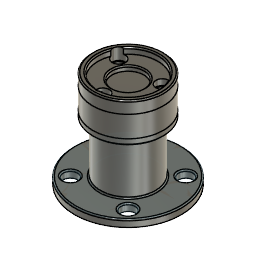
RV1-WHL-001_Wheel_Hub_Adapter (Autodesk Fusion 360 design; units mm, degrees)
part number: 2026-03-30-19-50-54-064
Autodesk Fusion 360 part; units mm, degrees
note: some values were not read from the file. Set by a fixed rule: which sketch regions a step uses.
sketch "Sketch1" plane through (0, 0, 0) normal (0, 0, 1) x (1, 0, 0)
  circle A0 centre (0, 0) radius 45.25
  line L0 (24.5, -24.5) -> (-24.5, -24.5) construction
  line L1 (-24.5, -24.5) -> (-24.5, 24.5) construction
  line L2 (-24.5, 24.5) -> (24.5, 24.5) construction
  line L3 (24.5, 24.5) -> (24.5, -24.5) construction
  line L4 (24.5, -24.5) -> (-24.5, 24.5) construction
  line L5 (-24.5, -24.5) -> (24.5, 24.5) construction
  circle A1 centre (-24.5, 24.5) radius 6.15
  circle A2 centre (24.5, 24.5) radius 6.15
  circle A3 centre (-24.5, -24.5) radius 6.15
  circle A4 centre (24.5, -24.5) radius 6.15
  circle A5 centre (0, 0) radius 20.25
  dimension "d1" = 90.5
  dimension "d2" = 49
  dimension "d3" = 49
  dimension "d4" = 12.3
  dimension "d5" = 12.3
  dimension "d6" = 12.3
  dimension "d7" = 12.3
  dimension "d10" = 40.5
  constraint coincident A0.centre A5.centre
  constraint horizontal L0
  constraint perpendicular L0 L1
  constraint parallel L0 L2
  constraint parallel L1 L3
  constraint coincident L4 A0.centre
  constraint coincident L5 A0.centre
  constraint coincident L1.end L2.start
  constraint coincident L2.end L3.start
  constraint coincident L0.end L1.start
  constraint coincident L0.start L3.end
  measures "d1" diameter of A0
  measures "d2" distance of L1.end L2.end
  measures "d3" distance of L0.end L1.end
  measures "d4" diameter of A1
  measures "d5" diameter of A2
  measures "d6" diameter of A3
  measures "d7" diameter of A4
  measures "d10" diameter of A5
extrude "Extrude1" add sketch "Sketch1" along normal blind 6 makes body 1
sketch "Sketch2" plane through (0, 0, 6) normal (0, 0, 1) x (-1, 0, 0)
  circle A0 centre (24.5, 24.5) radius 6.15
  circle A1 centre (24.5, -24.5) radius 6.15
  circle A2 centre (-24.5, 24.5) radius 6.15
  circle A3 centre (-24.5, -24.5) radius 6.15
  circle A4 centre (0, 0) radius 20.25
  circle A5 centre (0, 0) radius 45.25
  circle A6 centre (0, 0) radius 23.4
  dimension "d11" = 46.8
  constraint coincident A4.centre A5.centre
  measures "d11" diameter of A6
extrude "Extrude2" add sketch "Sketch2" along normal blind 35.5 contours A6 bodies 1
sketch "Sketch3" plane through (0, 0, 41.5) normal (0, 0, 1) x (-1, 0, 0)
  circle A0 centre (0, 0) radius 20.25
  circle A1 centre (0, 0) radius 23.4
  circle A2 centre (0, 0) radius 23.6 construction
  circle A3 centre (0, 21.35) radius 5.5
  circle A4 centre (-18.4897, -10.675) radius 5.5
  circle A5 centre (18.4896, -10.675) radius 5.5
  circle A6 centre (0, 0) radius 30
  dimension "d14" = 47.2
  dimension "d15" = 11
  dimension "d20" = 360
  dimension "d21" = 21.35
  dimension "d22" = 60
  constraint coincident A0.centre A1.centre
  measures "d14" diameter of A2
  measures "d15" diameter of A3
  measures "d21" vertical distance of A0.centre A3.centre
  measures "d22" diameter of A6
extrude "Extrude3" add sketch "Sketch3" along normal blind 10 separate body contours A0 A3 A4 A5 | A0 A1 A3 A5 | A0 A1 A3 A4 | A0 A1 A4 A5 | A6 makes body 2
sketch "Sketch4" plane through (0, 0, 51.5) normal (0, 0, 1) x (-1, 0, 0)
  circle A0 centre (18.4896, -10.675) radius 5.5
  circle A1 centre (-18.4897, -10.675) radius 5.5
  circle A2 centre (0, 21.35) radius 5.5
  circle A3 centre (0, 0) radius 30
  circle A4 centre (0, 0) radius 25.5
  dimension "d25" = 51
  constraint coincident A3.centre A4.centre
  measures "d25" diameter of A4
extrude "Extrude4" cut sketch "Sketch4" against normal blind 5 contours A0 A4 | A0 A1 A2 A4 | A1 A4 | A2 A4 picked at (19.2783, -11.1304) picked at (-19.3262, -11.052) picked at (-0.0449, 22.2612) bodies 2
sketch "Sketch5" plane through (0, 0, 46.5) normal (0, 0, 1) x (-1, 0, 0)
  arc A0 (-19.8531, -16.0033) -> (19.853, -16.0034) centre (0, 0) ccw
  arc A1 (23.7858, -9.1916) -> (19.853, -16.0034) centre (18.4896, -10.675) ccw
  arc A2 (23.7858, -9.1916) -> (3.9328, 25.1949) centre (0, 0) ccw
  arc A3 (-3.9327, 25.1949) -> (3.9328, 25.1949) centre (0, 21.35) ccw
  arc A4 (-3.9327, 25.1949) -> (-23.7858, -9.1915) centre (0, 0) ccw
  arc A5 (-19.8531, -16.0033) -> (-23.7858, -9.1915) centre (-18.4897, -10.675) ccw
  circle A6 centre (0, 0) radius 13.5
  dimension "d28" = 27
  constraint coincident A0.centre A2.centre
  measures "d28" diameter of A6
extrude "Extrude5" cut sketch "Sketch5" against normal blind 4 contours A6 bodies 2
sketch "Sketch6" plane through (0, 0, 6) normal (0, 0, 1) x (-1, 0, 0)
  circle A0 centre (0, 0) radius 23.4
  circle A1 centre (24.5, -24.5) radius 6.15
  circle A2 centre (-24.5, -24.5) radius 6.15
  circle A3 centre (-24.5, 24.5) radius 6.15
  circle A4 centre (24.5, 24.5) radius 6.15
  circle A5 centre (0, 0) radius 45.25
move_body "Move1" bodies 2 to x (1, 0, 0) y (0, 1, 0) z (0, 0, 1) at (0, 0, 31)
extrude "Extrude6" add 1 faces at (-22.1875, 2.1686, 41.5) along direction (0, 0, 1) blind 7 on bodies 1 bodies 1
sketch "Sketch7" plane through (0, 0, 48.5) normal (0, 0, 1) x (-1, 0, 0)
  circle A0 centre (0, 0) radius 20.25
  circle A1 centre (0, 0) radius 23.4
  circle A2 centre (0, 0) radius 23.4
  constraint coincident A0.centre A1.centre
extrude "Extrude7" add sketch "Sketch7" along normal blind 4 and the other way blind 0.5 contours A0 | A1 A2 bodies 1
sketch "Sketch8" plane through (0, 0, 72.5) normal (0, 0, -1) x (1, 0, 0)
  circle A0 centre (-18.4896, -10.675) radius 5.5
  circle A1 centre (0, 21.35) radius 5.5
  circle A2 centre (18.4897, -10.675) radius 5.5
  circle A3 centre (0, 0) radius 30
  circle A4 centre (0, 0) radius 30
  constraint coincident A3.centre A4.centre
extrude "Extrude8" add sketch "Sketch8" along normal blind 18 separate body contours A0 | A1 | A2 | A3 A4 makes body 3
sketch "Sketch9" plane through (0, 0, 77.5) normal (0, 0, 1) x (-1, 0, 0)
  circle A0 centre (0, 0) radius 13.5
  arc A1 (-19.8531, -16.0033) -> (19.853, -16.0034) centre (0, 0) ccw
  arc A2 (23.7858, -9.1916) -> (19.853, -16.0034) centre (18.4896, -10.675) ccw
  arc A3 (23.7858, -9.1916) -> (3.9328, 25.1949) centre (0, 0) ccw
  arc A4 (-3.9327, 25.1949) -> (3.9328, 25.1949) centre (0, 21.35) ccw
  arc A5 (-3.9327, 25.1949) -> (-23.7858, -9.1915) centre (0, 0) ccw
  arc A6 (-19.8531, -16.0033) -> (-23.7858, -9.1915) centre (-18.4897, -10.675) ccw
  circle A7 centre (0, 21.35) radius 4.4
  circle A8 centre (-18.4897, -10.675) radius 4.4
  circle A9 centre (18.4896, -10.675) radius 4.4
  dimension "d41" = 8.8
  dimension "d42" = 8.8
  dimension "d43" = 8.8
  constraint concentric A4 A7
  constraint concentric A6 A8
  constraint concentric A2 A9
  measures "d41" diameter of A7
  measures "d42" diameter of A8
  measures "d43" diameter of A9
extrude "Extrude9" cut sketch "Sketch9" against normal blind 18.8908 contours A7 | A8 | A9 bodies 3
extrude "Extrude10" add 1 faces at (7.6631, -11.2397, 54.5) along direction (0, 0, -1) blind 5 separate body on bodies 3 makes body 4
fillet "Fillet1" radius 1 7 edges at (-18.8796, 7.3227, 0) (27.9698, 10.8485, 82.5) (-22.0837, -12.75, 82.5) (22.0836, -12.75, 82.5) (0, 25.5, 82.5) (12.5864, -4.8818, 77.5) (-27.9698, 10.8485, 49.5) 1 faces at (-11.4117, -31.3657, 6) on bodies 1 2 4
